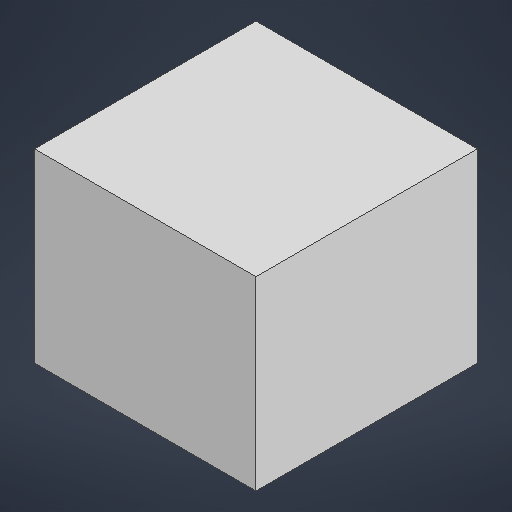
# Autodesk Inventor part: 前纸铲纸
Saved by Autodesk Inventor 2025 (Build 290162000, 162)
## iProperties
Created: 2026-04-23
Part Number: 前纸铲纸
Material: 常规
Document SubType Name: Modeling
Designer: XH
Density: 1 g/cm^3
Appearance: 默认
Author: XH
Autodesk Inventor part; units mm, degrees
ref_plane "YZ Plane" through (0, 0, 0) normal (1, 0, 0) x (0, 1, 0)
ref_plane "XZ Plane" through (0, 0, 0) normal (0, 1, 0) x (-1, 0, 0)
ref_plane "XY Plane" through (0, 0, 0) normal (0, 0, 1) x (1, 0, 0)
sketch "草图1" plane through (0, 0, 0) normal (0, 0, 1) x (1, 0, 0)
  line L0 (5, -4.1908) -> (-5, -4.1908)
  line L1 (-5, -4.1908) -> (-5, 4.1908)
  line L2 (-5, 4.1908) -> (5, 4.1908)
  line L3 (5, 4.1908) -> (5, -4.1908)
  line L4 (5, -4.1908) -> (-5, 4.1908) construction
  line L5 (-5, -4.1908) -> (5, 4.1908) construction
  point P0 (0, 0)
  dimension "d0" = 10
  constraints: 12 end point, 2 midpoint, 2 parallel, 1 horizontal, 1 perpendicular
  measures "d0" distance of L1.end L2.end
extrude "拉伸1" add sketch "草图1" along normal blind 10
